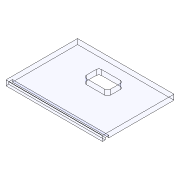
# Autodesk Inventor part: Lidar Sensor Case 4 v2
Saved by Autodesk Inventor 2018.3 (Build 223284000, 284)
## iProperties
Created: 2019-03-08
Part Number: Lidar Sensor Case 4 v2
Material: Generic
Document SubType Name: Modeling
Designer: aye06091
Mass: 6.36624 g
Surface Area: 51.9068 cm^2
Volume: 6.36624 cm^3
Density: 1 g/cm^3
Appearance: Clear - Blue
Author: aye06091
Autodesk Inventor part; units mm, degrees
ref_plane "YZ Plane" through (0, 0, 0) normal (1, 0, 0) x (0, 1, 0)
ref_plane "XZ Plane" through (0, 0, 0) normal (0, 1, 0) x (-1, 0, 0)
ref_plane "XY Plane" through (0, 0, 0) normal (0, 0, 1) x (1, 0, 0)
sketch "Sketch1" plane through (0, 0, 0) normal (0, 1, 0) x (-1, 0, 0)
  line L0 (0, 0) -> (-55.626, 0)
  line L1 (-55.626, 0) -> (-55.626, 41.275)
  line L2 (-55.626, 41.275) -> (0, 41.275)
  line L3 (0, 41.275) -> (0, 0)
  dimension "d0" = 41.275
  dimension "d1" = 55.626
  constraints: 8 end point, 2 parallel, 1 horizontal, 1 perpendicular
  measures "d0" distance of L2.end L0.start
  measures "d1" distance of L0.start L0.end
extrude "Extrusion1" add sketch "Sketch1" against normal blind 2.9972
sketch "Sketch2" plane through (0, 0, 0) normal (0, 1, 0) x (1, 0, 0)
  line L0 (0, -41.275) -> (0, 0) projected
  line L1 (55.626, -41.275) -> (0, -41.275) projected
  line L2 (20.828, -8.5725) -> (34.798, -8.5725)
  line L3 (34.798, -8.5725) -> (34.798, -17.4625)
  line L4 (34.798, -17.4625) -> (20.828, -17.4625)
  line L5 (20.828, -17.4625) -> (20.828, -8.5725)
  line L6 (55.626, 0) -> (55.626, -41.275) projected
  point P0 (27.813, -13.0175)
  dimension "d7" = 8.89
  dimension "d17" = 13.97
  dimension "d22" = 6.985
  dimension "d23" = 4.445
  dimension "d24" = 27.813
  dimension "d25" = 27.813
  dimension "d26" = 28.2575
  constraints: 8 end point, 2 parallel, 1 horizontal, 1 perpendicular
  measures "d7" distance of L2.end L3.end
  measures "d17" distance of L2.start L2.end
  measures "d22" distance from line of L5 point (27.813, -13.017)
  measures "d23" distance from line of L4 point (27.813, -13.017)
  measures "d24" distance from line of L0 point (27.813, -13.017)
  measures "d25" distance from line of L6 point (27.813, -13.017)
  measures "d26" distance from line of L1 point (27.813, -13.017)
extrude "Extrusion2" cut sketch "Sketch2" against normal blind 2.9972
fillet "Fillet1" radius 1.5875 4 edges at (20.828, -1.4986, 8.5725) (20.828, -1.4986, 17.4625) (34.798, -1.4986, 17.4625) (34.798, -1.4986, 8.5725)
sketch "Sketch6" plane through (0, -2.9972, 0) normal (0, -1, 0) x (1, 0, 0)
  line L0 (55.626, 0) -> (55.626, 41.275) projected
  line L1 (55.626, 41.275) -> (0, 41.275) projected
  line L2 (0, 41.275) -> (0, 0) projected
  line L3 (55.626, 39.6875) -> (0, 39.6875)
  line L4 (0, 39.6875) -> (0, 37.5285)
  line L5 (0, 37.5285) -> (55.626, 37.5285)
  line L6 (55.626, 37.5285) -> (55.626, 39.6875)
  dimension "d31" = 1.5875
  dimension "d32" = 2.159
  constraints: 8 end point, 2 parallel, 2 point on line, 1 horizontal, 1 perpendicular
  measures "d31" distance between parallel lines of L1 L3
  measures "d32" distance between parallel lines of L5 L3
extrude "Extrusion6" cut sketch "Sketch6" against normal blind 1.2446 contours L5 L2 L3 L0
body "Solid1"
